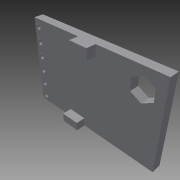
# Autodesk Inventor part: polyhexpart
Saved by Autodesk Inventor 2015 SP1 (Build 190203100, 203)
## iProperties
Created: 2015-04-18
Part Number: polyhexpart
Material: Generic
Document SubType Name: Modeling
Designer: Lab User
Density: 1 g/cm^3
Appearance: Default
Author: Lab User
Autodesk Inventor part; units mm, degrees
ref_plane "YZ Plane" through (0, 0, 0) normal (1, 0, 0) x (0, 1, 0)
ref_plane "XZ Plane" through (0, 0, 0) normal (0, 1, 0) x (-1, 0, 0)
ref_plane "XY Plane" through (0, 0, 0) normal (0, 0, 1) x (1, 0, 0)
sketch "Sketch2" plane through (0, 0, 0) normal (0, 0, 1) x (1, 0, 0)
  line L0 (-36.8686, 26.7016) -> (-30.1114, 30.7457)
  line L1 (-30.1114, 30.7457) -> (-23.2304, 26.9158)
  line L2 (-23.2304, 26.9158) -> (-23.1068, 19.0418)
  line L3 (-23.1068, 19.0418) -> (-29.864, 14.9977)
  line L4 (-29.864, 14.9977) -> (-36.7449, 18.8276)
  line L5 (-36.7449, 18.8276) -> (-36.8686, 26.7016)
  line L6 (-111.0137, 35.5717) -> (-17.2877, 35.5717)
  line L7 (-17.2877, 35.5717) -> (-17.2877, -24.1183)
  line L8 (-17.2877, -24.1183) -> (-111.0137, -24.1183)
  line L9 (-111.0137, -24.1183) -> (-111.0137, 35.5717)
  line L10 (-101.137, 28.7391) -> (-70.6621, 28.7391)
  line L11 (-70.6621, 28.7391) -> (-70.6621, -18.2509)
  line L12 (-70.6621, -18.2509) -> (-101.137, -18.2509)
  line L13 (-101.137, -18.2509) -> (-101.137, 28.7391)
  point P0 (0, 0)
  point P1 (-29.9877, 22.8717)
  dimension "d1" = 7.874
  dimension "d3" = 59.69
  dimension "d5" = 12.7
  dimension "d6" = 93.726
  dimension "d39" = 46.99
  dimension "d41" = 6.8326
  dimension "d42" = 5.8674
  dimension "d43" = 12.7
  constraints: 28 end point, 4 parallel, 2 horizontal, 2 perpendicular, 13 other
  measures "d1" vertical distance of L1.end L2.end
  measures "d3" distance of L8.end L6.start
  measures "d5" distance from line of L7 point (-29.988, 22.872)
  measures "d6" distance of L6.start L6.end
  measures "d39" distance of L10.end L11.end
  measures "d41" distance between parallel lines of L6 L10
  measures "d42" distance between parallel lines of L8 L12
  measures "d43" distance from line of L6 point (-29.988, 22.872)
extrude "Extrusion1" add sketch "Sketch2" along normal blind 6.35 contours L6 L7 L8 L9 | L10 L11 L12 L13
sketch "Sketch3" plane through (0, 0, 6.35) normal (0, 0, 1) x (1, 0, 0)
  circle A0 centre (-107.8387, 30.4917) radius 1.905
  line L0 (-17.2877, 35.5717) -> (-111.0137, 35.5717) projected
  line L1 (-111.0137, 35.5717) -> (-111.0137, -24.1183) projected
  circle A1 centre (-107.8387, 20.3317) radius 1.905
  circle A2 centre (-107.8387, -10.1483) radius 1.905
  circle A3 centre (-107.8387, -20.3083) radius 1.905
  line L2 (-111.0137, -24.1183) -> (-17.2877, -24.1183) projected
  circle A4 centre (-107.8387, 10.1717) radius 1.905
  circle A5 centre (-107.8387, 0.0117) radius 1.905
  point P0 (0, 0)
  dimension "d9" = 3.81
  dimension "d10" = 5.08
  dimension "d11" = 3.175
  dimension "d13" = 3.81
  dimension "d14" = 3.81
  dimension "d15" = 3.81
  dimension "d17" = 3.175
  dimension "d18" = 3.175
  dimension "d19" = 3.175
  dimension "d21" = 10.16
  dimension "d24" = 3.81
  dimension "d25" = 3.81
  dimension "d26" = 3.175
  dimension "d27" = 3.175
  dimension "d28" = 10.16
  dimension "d29" = 10.16
  dimension "d33" = 10.16
  dimension "d44" = 10.16
  constraints: 6 centre point
  measures "d9" diameter of A0
  measures "d10" distance from line of A0.centre L0
  measures "d11" distance from line of A0.centre L1
  measures "d13" diameter of A1
  measures "d14" diameter of A2
  measures "d15" diameter of A3
  measures "d17" distance from line of L1 A1.centre
  measures "d18" distance from line of L1 A2.centre
  measures "d19" distance from line of L1 A3.centre
  measures "d21" distance of A3.centre A2.centre
  measures "d24" diameter of A4
  measures "d25" diameter of A5
  measures "d26" distance from line of L1 A5.centre
  measures "d27" distance from line of L1 A4.centre
  measures "d28" distance of A4.centre A1.centre
  measures "d29" distance of A4.centre A5.centre
  measures "d33" distance of A0.centre A1.centre
  measures "d44" distance of A2.centre A5.centre
extrude "Extrusion2" cut sketch "Sketch3" against normal blind 3.81
sketch "Sketch4" plane through (0, 0, 6.35) normal (0, 0, 1) x (1, 0, 0)
  line L0 (-17.2877, 35.5717) -> (-111.0137, 35.5717) projected
  line L1 (-72.9137, 35.5717) -> (-60.2137, 35.5717)
  line L2 (-60.2137, 35.5717) -> (-60.2137, 35.0891)
  line L3 (-60.2137, 35.0891) -> (-72.9137, 35.0891)
  line L4 (-72.9137, 35.0891) -> (-72.9137, 35.5717)
  line L5 (-111.0137, -24.1183) -> (-17.2877, -24.1183) projected
  line L6 (-111.0137, 35.5717) -> (-111.0137, -24.1183) projected
  line L7 (-72.9137, 35.5717) -> (-60.2137, 35.5717)
  line L8 (-60.2137, 35.5717) -> (-60.2137, 28.7391)
  line L9 (-60.2137, 28.7391) -> (-72.9137, 28.7391)
  line L10 (-72.9137, 28.7391) -> (-72.9137, 35.5717)
  line L11 (-69.1037, -24.1183) -> (-81.8037, -24.1183)
  line L12 (-81.8037, -24.1183) -> (-81.8037, -18.1493)
  line L13 (-81.8037, -18.1493) -> (-69.1037, -18.1493)
  line L14 (-69.1037, -18.1493) -> (-69.1037, -24.1183)
  point P0 (0, 0)
  dimension "d34" = 59.2074
  dimension "d35" = 12.7
  dimension "d36" = 38.1
  dimension "d45" = 6.8326
  dimension "d46" = 12.7
  dimension "d47" = 5.969
  dimension "d48" = 29.21
  constraints: 24 end point, 6 parallel, 3 horizontal, 3 perpendicular, 2 point on line
  measures "d34" distance between parallel lines of L5 L3
  measures "d35" distance between parallel lines of L4 L2
  measures "d36" distance between parallel lines of L6 L4
  measures "d45" distance between parallel lines of L0 L9
  measures "d46" distance between parallel lines of L12 L14
  measures "d47" distance between parallel lines of L11 L13
  measures "d48" distance between parallel lines of L6 L12
extrude "Extrusion3" add sketch "Sketch4" along normal blind 6.35
body "Solid1"
